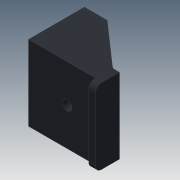
# Autodesk Inventor part: FLUGGER TRAY UPSTOP FLAP 
Saved by Autodesk Inventor 2020.3 (Build 243373000, 373)
## iProperties
RuleStatus: InUse
AfterDocSave0: file://Part Number Cleaner
Created: 2019-11-18
Material: ABS, BLACK
Vendor: HHMI: JRC - ID&F
Document SubType Name: Modeling
Designer: arnoldj
Density: 1.06 g/cm^3
Appearance: Black Anodize
DESIGN DEPARTMENT: HHMI: JRC - ID&F
ALTERED ITEM PART NUMBER: N/A
ALTERED ITEM VENDOR: N/A
ALTERED ITEM DESCRIPTION: N/A
Author: arnoldj
Revision Number: 0
Autodesk Inventor part; units mm, degrees
ref_plane "YZ Plane" through (0, 0, 0) normal (1, 0, 0) x (0, 1, 0)
ref_plane "XZ Plane" through (0, 0, 0) normal (0, 1, 0) x (-1, 0, 0)
ref_plane "XY Plane" through (0, 0, 0) normal (0, 0, 1) x (1, 0, 0)
sketch "Sketch1" plane through (0, 0, 0) normal (0, 1, 0) x (-1, 0, 0)
  line L0 (0, -37.4904) -> (0, 6.2484) projected
  line L1 (-44.958, 0) -> (7.493, 0) projected
  line L2 (0, 0) -> (-37.465, 0)
  line L3 (-37.465, 0) -> (-37.465, -9.525)
  line L4 (-37.465, -9.525) -> (0, -9.525)
  line L5 (0, -9.525) -> (0, 0)
  line L6 (0, -9.525) -> (-12.7, -9.525)
  line L7 (-12.7, -9.525) -> (-12.7, -31.242)
  line L8 (0, -31.242) -> (0, -9.525)
  line L9 (0, -31.242) -> (-12.7, -31.242)
  dimension "d10" = 9.525
  dimension "d36" = 31.242
  dimension "d37" = 12.7
  dimension "d38" = 37.465
  constraints: 16 end point, 3 parallel, 3 perpendicular, 2 horizontal, 2 point on line
  measures "d10" distance of L2.end L3.end
  measures "d36" distance between parallel lines of L9 L1
  measures "d37" distance of L8.start L7.end
  measures "d38" distance between parallel lines of L0 L3
extrude "Extrusion3" add sketch "Sketch1" along normal mid plane 41.91
sketch "Sketch2" plane through (37.465, 20.955, -9.525) normal (0, 0, -1) x (-1, 0, 0)
  line L0 (24.765, -41.91) -> (24.765, 0) projected
  line L1 (0, 0) -> (24.765, 0) projected
  line L2 (0, -41.91) -> (0, 0) projected
  line L3 (24.765, -41.91) -> (0, -41.91) projected
  line L4 (-7.493, -20.955) -> (44.958, -20.955) projected
  line L5 (37.465, -41.91) -> (37.465, 0) projected
  point P0 (37.465, -20.955)
  point P1 (15.875, -20.955)
  dimension "d56" = 0
  dimension "d57" = 21.59
  measures "d56" distance from line of L4 point (15.875, -20.955)
  measures "d57" distance from line of L5 point (15.875, -20.955)
hole "Hole1" at (21.59, 0, -9.525) direction (0, 0, 1) diameter 5.5118 end through all clearance for "Socket Head Cap Screw" size "M5" standard "Ansi Metric M Profile"
sketch "Sketch3" plane through (0, -20.955, 0) normal (0, 1, 0) x (-1, 0, 0)
  line L0 (-12.7, -31.242) -> (-12.7, -9.525) projected
  line L1 (-12.7, -9.525) -> (-37.465, -9.525) projected
  line L2 (-37.465, -9.525) -> (-12.7, -31.242)
  line L3 (-12.7, -31.242) -> (-12.7, -9.525)
  line L4 (-37.465, -9.525) -> (-12.7, -9.525)
  point P0 (0, 0)
  constraints: 6 end point, 1 horizontal, 1 vertical
extrude "Extrusion4" add sketch "Sketch3" along normal blind 6.35
sketch "Sketch4" plane through (12.7, 20.955, -31.242) normal (0, 0, -1) x (-1, 0, 0)
  line L0 (12.7, -50.292) -> (12.7, 8.382) projected
  line L1 (-32.258, -20.955) -> (20.193, -20.955) projected
  line L2 (0, -35.56) -> (0, 0) projected
  point P0 (12.7, -20.955)
  point P1 (6.35, -9.525)
  point P2 (6.35, -32.385)
  point P3 (6.35, -20.955)
  dimension "d39" = 11.43
  dimension "d40" = 11.43
  dimension "d41" = 6.35
  dimension "d63" = 12.7
  constraints: 2 vertical alignment, 1 point on line
  measures "d39" distance from line of point (6.35, -9.525) L1
  measures "d40" distance from line of L1 point (6.35, -32.385)
  measures "d41" distance from line of point (6.35, -9.525) L0
  measures "d63" distance between parallel lines of L0 L2
hole "Hole2" at (6.35, 11.43, -31.242) at (6.35, -11.43, -31.242) at (6.35, 0, -31.242) direction (0, 0, 1) diameter 2.4384 depth 10.16 tip angle 118 clearance for "Flat Head Machine Screw (100)" size "#2" standard "Ansi Unified Screw Threads"
sketch "Sketch5" plane through (12.7, 20.955, -9.525) normal (1, 0, 0) x (0, 0, -1)
  line L0 (-15.7734, -20.955) -> (27.9654, -20.955) projected
  line L1 (-9.525, -50.292) -> (-9.525, 8.382) projected
  line L2 (14.097, -12.0015) -> (15.875, -12.0015)
  line L3 (15.875, -12.0015) -> (15.875, -7.0485)
  line L4 (15.875, -7.0485) -> (14.097, -7.0485)
  line L5 (14.097, -7.0485) -> (14.097, -12.0015)
  line L6 (14.097, -12.0015) -> (15.875, -7.0485) construction
  line L7 (15.875, -12.0015) -> (14.097, -7.0485) construction
  line L8 (14.097, -23.4315) -> (15.875, -23.4315)
  line L9 (15.875, -23.4315) -> (15.875, -18.4785)
  line L10 (15.875, -18.4785) -> (14.097, -18.4785)
  line L11 (14.097, -18.4785) -> (14.097, -23.4315)
  line L12 (14.097, -23.4315) -> (15.875, -18.4785) construction
  line L13 (15.875, -23.4315) -> (14.097, -18.4785) construction
  line L14 (14.097, -34.8615) -> (15.875, -34.8615)
  line L15 (15.875, -34.8615) -> (15.875, -29.9085)
  line L16 (15.875, -29.9085) -> (14.097, -29.9085)
  line L17 (14.097, -29.9085) -> (14.097, -34.8615)
  line L18 (14.097, -34.8615) -> (15.875, -29.9085) construction
  line L19 (15.875, -34.8615) -> (14.097, -29.9085) construction
  line L20 (21.717, -35.56) -> (21.717, 0) projected
  point P0 (-9.525, -20.955)
  point P1 (14.986, -9.525)
  point P2 (14.986, -20.955)
  point P3 (14.986, -32.385)
  point P4 (14.986, -9.525)
  point P5 (14.986, -32.385)
  dimension "d49" = 4.953
  dimension "d50" = 1.778
  dimension "d51" = 11.43
  dimension "d58" = 7.62
  dimension "d59" = 11.43
  constraints: 36 end point, 8 midpoint, 6 parallel, 4 equal length, 3 horizontal, 3 perpendicular, 2 point on line, 1 vertical alignment
  measures "d49" distance of L2.end L3.end
  measures "d50" distance of L3.end L4.end
  measures "d51" distance from line of L0 point (14.986, -9.525)
  measures "d58" distance between parallel lines of L20 L5
  measures "d59" distance from line of L0 point (14.986, -32.385)
extrude "Extrusion5" cut sketch "Sketch5" along normal blind 10.16 and the other way blind 8.89
sketch "Sketch6" plane through (0, 20.955, 0) normal (0, 1, 0) x (1, 0, 0)
  line L0 (12.7, 9.525) -> (12.7, 31.242) projected
  line L1 (37.465, 9.525) -> (12.7, 9.525) projected
  line L2 (37.465, 9.525) -> (12.7, 31.242) projected
  point P0 (0, 0)
extrude "Extrusion6" add sketch "Sketch6" against normal blind 6.35
sketch "Sketch7" plane through (0, 20.955, 0) normal (0, 1, 0) x (1, 0, 0)
  line L0 (0, 0) -> (37.465, 0) projected
  line L1 (37.465, 0) -> (37.465, 9.525) projected
  line L2 (25.7746, 0) -> (37.5697, -3.1605)
  line L3 (37.5697, -3.1605) -> (37.465, 0)
  line L4 (25.7746, 0) -> (37.465, 0)
  dimension "d64" = 11.684
  dimension "d65" = 15
  constraints: 6 end point, 1 horizontal, 1 point on line
  measures "d64" distance from line of L2.start L3
  measures "d65" angle of L0 L2
extrude "Extrusion7" [suppressed]
sketch "Sketch8" plane through (37.465, -20.955, 0) normal (1, 0, 0) x (0, 0, -1)
  line L0 (9.525, 0) -> (9.525, 6.35) projected
  line L1 (9.525, 6.35) -> (9.525, 35.56) projected
  line L2 (9.525, 35.56) -> (9.525, 41.91) projected
  line L3 (0, 41.91) -> (9.525, 41.91) projected
  line L4 (0, 0) -> (0, 41.91) projected
  line L5 (9.525, 0) -> (0, 0) projected
  line L6 (9.525, 41.91) -> (-3.81, 41.91)
  line L7 (-3.81, 41.91) -> (-3.81, 0)
  line L8 (-3.81, 0) -> (9.525, 0)
  line L9 (9.525, 0) -> (9.525, 41.91)
  point P0 (0, 20.955)
  dimension "d68" = 0
  dimension "d69" = 3.81
  constraints: 8 end point, 2 parallel, 1 horizontal, 1 perpendicular
  measures "d68" distance between parallel lines of L5 L8
  measures "d69" distance between parallel lines of L4 L7
extrude "Extrusion8" add sketch "Sketch8" along normal blind 3.81
fillet "Fillet2" radius 3.175 4 edges at (37.465, 17.78, -9.525) (37.465, -17.78, -9.525) (39.37, 20.955, 3.81) (39.37, -20.955, 3.81)
equation "\"d40\" = d39"
equation "\"d41\" = 0.5 * d63"
body "Solid2"
